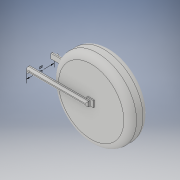
# Autodesk Inventor part: rearWheel
Saved by Autodesk Inventor 2018 (Build 220112000, 112)
## iProperties
Created: 2018-02-23
Part Number: rearWheel
Material: Generic
Document SubType Name: Modeling
Designer: rochee19
Density: 1 g/cm^3
Appearance: Default
Author: rochee19
Autodesk Inventor part; units mm, degrees
ref_plane "YZ Plane" through (0, 0, 0) normal (1, 0, 0) x (0, 1, 0)
ref_plane "XZ Plane" through (0, 0, 0) normal (0, 1, 0) x (-1, 0, 0)
ref_plane "XY Plane" through (0, 0, 0) normal (0, 0, 1) x (1, 0, 0)
sketch "Sketch1" plane through (0, 0, 0) normal (0, 0, 1) x (1, 0, 0)
  circle A0 centre (0, 0) radius 311.15
  dimension "d0" = 622.3
  constraints: 1 centre point, 1 coincident
  measures "d0" diameter of A0
extrude "Extrusion1" add sketch "Sketch1" along normal blind 152.4
sketch "Sketch2" plane through (0, 0, 152.4) normal (0, 0, 1) x (1, 0, 0)
  line L0 (-25.4, -25.4) -> (25.4, -25.4)
  line L1 (25.4, -25.4) -> (25.4, 25.4)
  line L2 (25.4, 25.4) -> (-25.4, 25.4)
  line L3 (-25.4, 25.4) -> (-25.4, -25.4)
  line L4 (-25.4, -25.4) -> (25.4, 25.4) construction
  line L5 (25.4, -25.4) -> (-25.4, 25.4) construction
  point P0 (0, 0)
  dimension "d3" = 50.8
  dimension "d4" = 50.8
  constraints: 12 end point, 2 midpoint, 2 parallel, 1 horizontal, 1 perpendicular
  measures "d3" distance of L2.end L1.end
  measures "d4" distance of L1.end L0.end
extrude "Extrusion6" add sketch "Sketch2" along normal blind 8.4667
sketch "Sketch7" plane through (0, 0, 160.8667) normal (0, 0, 1) x (1, 0, 0)
  line L0 (-25.4, -25.4) -> (25.4, -25.4) projected
  line L1 (0, -25.4) -> (-482.6, -25.4)
  line L2 (-482.6, -25.4) -> (-482.6, 12.7)
  line L3 (-482.6, 12.7) -> (0, 12.7)
  line L4 (0, 12.7) -> (0, -25.4)
  point P0 (0, 0)
  dimension "d23" = 482.6
  dimension "d24" = 38.1
  constraints: 8 end point, 2 parallel, 1 collinear, 1 midpoint, 1 perpendicular
  measures "d23" distance of L1.start L1.end
  measures "d24" distance of L1.end L2.end
extrude "Extrusion7" add sketch "Sketch7" along normal blind 25.4
sketch "Sketch8" plane through (0, 0, 0) normal (0, 0, -1) x (-1, 0, 0)
  line L0 (-25.4, -25.4) -> (-25.4, 25.4) projected
  line L1 (25.4, -25.4) -> (-25.4, -25.4)
  line L2 (-25.4, -25.4) -> (-25.4, 25.4)
  line L3 (-25.4, 25.4) -> (25.4, 25.4)
  line L4 (25.4, 25.4) -> (25.4, -25.4)
  line L5 (25.4, -25.4) -> (-25.4, 25.4) construction
  line L6 (-25.4, -25.4) -> (25.4, 25.4) construction
  point P0 (0, 0)
  constraints: 12 end point, 2 midpoint, 2 parallel, 1 horizontal, 1 perpendicular
extrude "Extrusion8" add sketch "Sketch8" along normal blind 8.4667
sketch "Sketch9" plane through (0, 0, -8.4667) normal (0, 0, -1) x (-1, 0, 0)
  point P0 (0, 0)
sketch "Sketch10" plane through (0, 0, -8.4667) normal (0, 0, -1) x (-1, 0, 0)
  line L0 (0, -25.4) -> (-25.4, -25.4) projected
  line L1 (482.6, 12.7) -> (482.6, -25.4) projected
  line L2 (0, -25.4) -> (482.6, -25.4)
  line L3 (482.6, -25.4) -> (482.6, 12.7)
  line L4 (482.6, 12.7) -> (0, 12.7)
  line L5 (0, 12.7) -> (0, -25.4)
  point P0 (0, 0)
  constraints: 8 end point, 2 parallel, 1 horizontal, 1 perpendicular
extrude "Extrusion9" add sketch "Sketch10" along normal blind 25.4
sketch "Sketch12" plane through (0, 0, 186.2667) normal (0, 0, 1) x (1, 0, 0)
  line L0 (-482.6, -25.4) -> (-482.6, 12.7) projected
  line L1 (0, -25.4) -> (-482.6, -25.4) projected
  line L2 (-482.6, 12.7) -> (-444.5, 12.7)
  line L3 (-444.5, 12.7) -> (-444.5, -25.4)
  line L4 (-444.5, -25.4) -> (-482.6, -25.4)
  line L5 (-482.6, -25.4) -> (-482.6, 12.7)
  circle A0 centre (-463.55, -6.35) radius 8.128
  point P0 (0, 0)
  dimension "d38" = 38.1
  dimension "d39" = 16.256
  constraints: 8 end point, 2 parallel, 1 centre point, 1 horizontal, 1 perpendicular, 1 point on line
  measures "d38" distance of L3.end L4.end
  measures "d39" diameter of A0
extrude "Extrusion11" add sketch "Sketch12" along normal blind 50.8 contours A0
sketch "Sketch13" plane through (-463.55, -6.35, 237.0667) normal (0, 0, 1) x (1, 0, 0)
  circle A0 centre (0, 0) radius 8.128
  point P0 (463.55, 6.35)
  constraints: 1 centre point
extrude "Extrusion12" cut sketch "Sketch13" against normal blind 25.4
sketch "Sketch14" plane through (-463.55, -6.35, 211.6667) normal (0, 0, 1) x (1, 0, 0)
  circle A0 centre (0, 0) radius 8.128
  point P0 (463.55, 6.35)
  constraints: 1 centre point
extrude "Extrusion13" add sketch "Sketch14" along normal blind 12.7
sketch "Sketch15" plane through (-463.55, -6.35, 224.3667) normal (0, 0, 1) x (1, 0, 0)
  circle A0 centre (0, 0) radius 8.128
  point P0 (463.55, 6.35)
  constraints: 1 centre point
extrude "Extrusion14" add sketch "Sketch15" along normal blind 6.35
sketch "Sketch16" plane through (-463.55, -6.35, 230.7167) normal (0, 0, 1) x (1, 0, 0)
  circle A0 centre (0, 0) radius 8.128
  point P0 (463.55, 6.35)
  constraints: 1 centre point
extrude "Extrusion15" add sketch "Sketch16" along normal blind 3.175
fillet "Fillet1" radius 50.8 2 edges at (-311.15, 0, 152.4) (-311.15, 0, 0)
fillet "Fillet2" radius 15.24 6 edges at (-241.3, 12.7, 186.2667) (-241.3, -25.4, 186.2667) (-241.3, 12.7, -33.8667) (-241.3, -25.4, -33.8667) (0, -6.35, -33.8667) (0, -6.35, 186.2667)
sketch "Sketch17" plane through (-463.55, -6.35, 233.8917) normal (0, 0, 1) x (1, 0, 0)
  circle A0 centre (0, 0) radius 8.128
  point P0 (463.55, 6.35)
  constraints: 1 centre point
extrude "Extrusion16" cut sketch "Sketch17" against normal blind 50.8
sketch "Sketch23" plane through (0, 0, 160.8667) normal (0, 0, -1) x (-1, 0, 0)
  line L0 (482.6, -25.4) -> (482.6, 12.7) projected
  line L1 (482.6, -6.35) -> (455.422, -6.35)
  arc A0 (456.3703, -2.54) -> (456.3703, -10.16) centre (463.55, -6.35) ccw projected
  circle A1 centre (463.55, -6.35) radius 8.128
  point P0 (0, 0)
  constraints: 2 end point, 1 centre point, 1 coincident, 1 horizontal, 1 midpoint, 1 point on circle
extrude "Extrusion20" add sketch "Sketch23" against normal blind 35.9918
sketch "Sketch24" plane through (0, 0, -8.4667) normal (0, 0, 1) x (1, 0, 0)
  line L0 (-482.6, -25.4) -> (-482.6, 12.7) projected
  line L1 (-482.6, -6.35) -> (-455.422, -6.35)
  circle A0 centre (-463.55, -6.35) radius 8.128 projected
  circle A1 centre (-463.55, -6.35) radius 8.128
  point P0 (0, 0)
  constraints: 2 end point, 1 centre point, 1 coincident, 1 horizontal, 1 horizontal alignment, 1 midpoint, 1 other
extrude "Extrusion21" add sketch "Sketch24" against normal blind 35.9918
body "Solid1"
